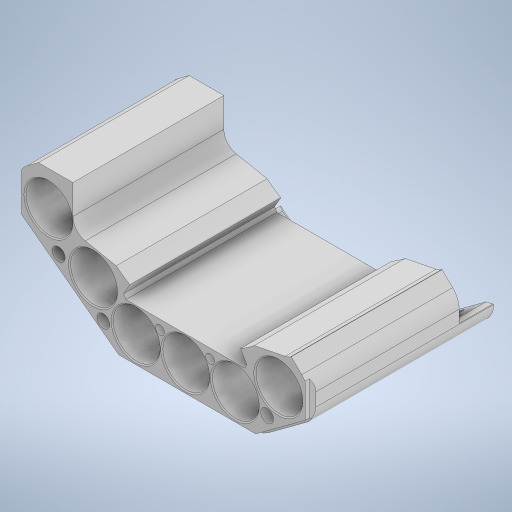
# Autodesk Inventor part: battery_mnt_right
Saved by Autodesk Inventor 2023.4 (Build 274418000, 418)
## iProperties
Created: 2024-01-27
Part Number: battery_mnt_right
Material: Generic
Document SubType Name: Modeling
Designer: aaron
Density: 1 g/cm^3
Appearance: Default
Author: aaron
Autodesk Inventor part; units mm, degrees
ref_plane "YZ Plane" through (0, 0, 0) normal (1, 0, 0) x (0, 1, 0)
ref_plane "XZ Plane" through (0, 0, 0) normal (0, 1, 0) x (-1, 0, 0)
ref_plane "XY Plane" through (0, 0, 0) normal (0, 0, 1) x (1, 0, 0)
sketch "Sketch1" plane through (0, 0, 0) normal (0, 0, 1) x (1, 0, 0)
  line L0 (28.444864, -49.267949) -> (27.444864, -51)
  line L1 (28.444864, -49.267949) -> (25.5, -44.167296)
  arc A0 (25.5, -44.167296) -> (38.751507, -33.156006) centre (0, 0) ccw
  arc A1 (38.751507, -33.156006) -> (51.999677, -30) centre (44.999677, -30) ccw
  line L2 (51.999677, 30) -> (51.999677, -30)
  arc A2 (51.999677, 30) -> (38.751507, 33.156006) centre (44.999677, 30) ccw
  arc A3 (38.751507, 33.156006) -> (25.5, 44.167296) centre (0, 0) ccw
  line L3 (25.5, 44.167296) -> (28.444864, 49.267949)
  line L4 (27.444864, 51) -> (28.444864, 49.267949)
  line L5 (27.444864, 51) -> (-27.444864, 51)
  line L6 (-28.444864, 49.267949) -> (-27.444864, 51)
  line L7 (-28.444864, 49.267949) -> (-25.5, 44.167296)
  arc A4 (-25.5, 44.167296) -> (-38.751507, 33.156006) centre (0, 0) ccw
  arc A5 (-38.751507, 33.156006) -> (-51.999677, 30) centre (-44.999677, 30) ccw
  line L8 (-51.999677, 30) -> (-51.999677, -30)
  arc A6 (-51.999677, -30) -> (-38.751507, -33.156006) centre (-44.999677, -30) ccw
  arc A7 (-38.751507, -33.156006) -> (-25.5, -44.167296) centre (0, 0) ccw
  line L9 (-25.5, -44.167296) -> (-28.444864, -49.267949)
  line L10 (-27.444864, -51) -> (-28.444864, -49.267949)
  line L11 (-27.444864, -51) -> (27.444864, -51)
  circle A8 centre (0, 0) radius 48
  circle A9 centre (44.999677, -30) radius 2.875
  circle A10 centre (44.999677, 30) radius 2.875
  circle A11 centre (-44.999677, 30) radius 2.875
  circle A12 centre (-44.999677, -30) radius 2.875
  line L12 (-43.944685, -76.472384) -> (38.141017, -76.472384)
  circle A13 centre (43.188005, -51) radius 10.85
  circle A14 centre (23, -63) radius 10.85
  circle A15 centre (0, -63) radius 10.85
  circle A16 centre (-23, -63) radius 10.85
  circle A17 centre (-63.495945, -32.562911) radius 10.85
  circle A18 centre (-42.787465, -50.133975) radius 10.85
  line L13 (-51.999677, -16.395024) -> (-68.142845, -16.395024)
  line L14 (57.082969, -58.824434) -> (57.082969, -43.439377)
  line L15 (57.082969, -43.439377) -> (49.113739, -35.663435)
  line L16 (-77.442937, -41.876031) -> (-31.413941, -76.472384)
  line L17 (57.082969, -58.824434) -> (33.195718, -76.472384)
  line L18 (-77.442937, -41.876031) -> (-77.442937, -23.26595)
  line L19 (-77.442937, -23.26595) -> (-68.142845, -16.395024)
  line L20 (-47.70661, -36.599635) -> (-27.043212, -40.695389)
  line L21 (0, 0) -> (0, -13.401061)
  line L22 (47.70661, -36.599635) -> (27.043212, -40.695389)
  point P0 (-43.377516, -36.809449)
  point P1 (43.377516, -36.809449)
  point P2 (-31.997646, -39.713356)
  point P3 (-46.360689, -36.866414)
  point P4 (46.360689, -36.866414)
  point P5 (31.997646, -39.713356)
  dimension "d2" = 21.7
  dimension "d3" = 21.7
  dimension "d4" = 21.7
  dimension "d5" = 21.7
  dimension "d6" = 21.7
  dimension "d7" = 21.7
  dimension "d12" = 96
  dimension "d13" = 54.88973
  dimension "d14" = 54.88973
  dimension "d15" = 60
  dimension "d16" = 60
  dimension "d17" = 7
  dimension "d18" = 7
  dimension "d19" = 51
  dimension "d20" = 51
  dimension "d21" = 12
  dimension "d22" = 12
  dimension "d23" = 12
  dimension "d24" = 23
  dimension "d25" = 0
  dimension "d26" = 23
  dimension "d28" = 102
  dimension "d29" = 51
  constraints: 46 end point, 19 centre point, 19 point on circle, 3 point on line, 2 symmetric about line, 2 vertical, 1 horizontal, 1 perpendicular, 1 tangent
  measures "d2" diameter of A13
  measures "d3" diameter of A14
  measures "d4" diameter of A15
  measures "d5" diameter of A16
  measures "d6" diameter of A17
  measures "d7" diameter of A18
  measures "d12" diameter of A8
  measures "d13" distance of L11.start L0.end
  measures "d14" distance of L5.start L6.end
  measures "d15" distance of L8.start L8.end
  measures "d16" distance of L2.start L2.end
  measures "d17" radius of A1
  measures "d18" radius of A6
  measures "d19" radius of A7
  measures "d20" radius of A0
  measures "d21" distance from line of A15.centre L11
  measures "d22" distance from line of L11 A14.centre
  measures "d23" distance from line of L11 A16.centre
  measures "d24" distance of A16.centre A15.centre
  measures "d25" horizontal distance of point (0, 0) A15.centre
  measures "d26" distance of A15.centre A14.centre
  measures "d28" distance between parallel lines of L5 L11
  measures "d29" distance from line of point (0, 0) L11
extrude "Extrusion1" add sketch "Sketch1" along normal blind 70 contours L1 A0 L22 A1 L15 L14 L17 L12 L16 L18 L19 L13 L8 A6 L20 A7 L9 L10 L11 L0
thicken "Thicken1" operation cut thickness 0.1 both sides no extend neighbours no toward (-1, 0, 0) faces at (-51.999677, -25.465008, 23.333333) (-51.022382, -33.567495, 46.666667) (-31.310695, -40.257178, 46.666667) (-27.463242, -47.567731, 23.333333) (-27.778197, -50.42265, 23.333333) (9.148288, -51, 23.333333) (28.11153, -49.845299, 23.333333) (26.481621, -45.867513, 23.333333) (31.310695, -40.257178, 23.333333) (48.836892, -35.854552, 23.333333) (-36.785327, -38.764375, 46.666667) (41.573008, -37.815395, 23.333333)
sketch "Sketch2" plane through (0, 0, 0) normal (0, 0, -1) x (-1, 0, 0)
  line L0 (-49.172511, -35.744341) -> (-49.113739, -35.663435)
  line L1 (-57.082969, -43.439377) -> (-49.113739, -35.663435)
  line L2 (-57.082969, -58.824434) -> (-57.082969, -43.439377)
  line L3 (-33.195718, -76.472384) -> (-57.082969, -58.824434)
  line L4 (31.413941, -76.472384) -> (-33.195718, -76.472384)
  line L5 (77.442937, -41.876031) -> (31.413941, -76.472384)
  line L6 (77.442937, -23.26595) -> (77.442937, -41.876031)
  line L7 (68.142845, -16.395024) -> (77.442937, -23.26595)
  line L8 (52.099677, -16.395024) -> (68.142845, -16.395024)
  line L9 (52.099677, -16.395024) -> (52.099677, -30)
  arc A0 (46.380132, -36.964506) -> (52.099677, -30) centre (44.999677, -30) ccw
  line L10 (46.380132, -36.964506) -> (32.041213, -39.806666)
  arc A1 (25.636554, -44.203813) -> (32.041213, -39.806666) centre (0, 0) ccw
  line L11 (25.636554, -44.203813) -> (28.560334, -49.267949)
  line L12 (28.560334, -49.267949) -> (27.502599, -51.1)
  line L13 (27.502599, -51.1) -> (-27.502599, -51.1)
  line L14 (-27.502599, -51.1) -> (-28.560334, -49.267949)
  line L15 (-28.560334, -49.267949) -> (-25.636554, -44.203813)
  arc A2 (-32.041213, -39.806666) -> (-25.636554, -44.203813) centre (0, 0) ccw
  line L16 (-32.041213, -39.806666) -> (-46.380132, -36.964506)
  arc A3 (-49.172511, -35.744341) -> (-46.380132, -36.964506) centre (-44.999677, -30) ccw
  circle A4 centre (0, -63) radius 10.85
  circle A5 centre (42.787465, -50.133975) radius 10.85
  circle A6 centre (63.495945, -32.562911) radius 10.85
  circle A7 centre (23, -63) radius 10.85
  circle A8 centre (-23, -63) radius 10.85
  circle A9 centre (-43.188005, -51) radius 10.85
  line L17 (-63.021311, -52.572205) -> (-32.701715, -74.972384)
  line L18 (-32.701715, -74.972384) -> (30.913077, -74.972384)
  line L19 (30.913077, -74.972384) -> (84.461316, -34.724411)
  line L20 (-33.195718, -76.472384) -> (-57.082969, -58.824434)
  line L21 (-55.582969, -67.648409) -> (-55.582969, -26.578043)
  line L22 (75.942937, -58.824434) -> (75.942937, -10.568938)
  point P0 (77.442937, -39.999571)
  point P1 (-57.082969, -56.959464)
  point P2 (75.942937, -22.157747)
  point P3 (75.942937, -41.127002)
  point P4 (-55.582969, -58.067667)
  point P5 (-55.582969, -41.975759)
  dimension "d30" = 1.5
  dimension "d32" = 1.5
  dimension "d33" = 1.5
  dimension "d50" = 1.5
  dimension "d51" = 1.5
  constraints: 10 end point, 2 vertical, 1 horizontal, 1 parallel
  measures "d30" distance between parallel lines of L4 L18
  measures "d32" distance between parallel lines of L3 L17
  measures "d33" distance between parallel lines of L5 L19
  measures "d50" distance between parallel lines of L6 L22
  measures "d51" distance between parallel lines of L2 L21
extrude "Extrusion2" cut sketch "Sketch2" against normal blind 2 contours L21 L17 L2 L1 | L21 L3 L2 L17 | L17 L18 L19 L22 L5 L4 L3 L21 | L22 L7 L6 L19 | L19 L6 L5 L22
sketch "Sketch3" plane through (0, 0, 0) normal (0, 0, -1) x (-1, 0, 0)
  circle A0 centre (38, -64.972384) radius 2.95
  circle A1 centre (-38, -64.972384) radius 2.95
  circle A2 centre (0, -63) radius 10.85
  line L0 (31.413941, -76.472384) -> (-33.195718, -76.472384)
  circle A3 centre (58.715512, -48.446115) radius 2.95
  line L1 (77.442937, -41.876031) -> (31.413941, -76.472384)
  point P0 (0, 0)
  dimension "d36" = 5.9
  dimension "d37" = 5.9
  dimension "d38" = 38
  dimension "d39" = 38
  dimension "d40" = 11.5
  dimension "d41" = 11.5
  dimension "d44" = 5.9
  dimension "d45" = 26.5
  dimension "d46" = 6
  constraints: 3 centre point
  measures "d36" diameter of A1
  measures "d37" diameter of A0
  measures "d38" horizontal distance of A1.centre A2.centre
  measures "d39" horizontal distance of A0.centre A2.centre
  measures "d40" distance from line of L0 A0.centre
  measures "d41" distance from line of L0 A1.centre
  measures "d44" diameter of A3
  measures "d45" distance of A0.centre A3.centre
  measures "d46" distance from line of L1 A3.centre
extrude "Extrusion3" cut sketch "Sketch3" against normal blind 15 contours A0 | A1 | A3
chamfer "Chamfer1" distance 1.5 angle 45 5 edges at (45.1393, -67.6484, 2) (0.8909, -76.4724, 2) (-54.4284, -59.1742, 2) (-77.4429, -32.571, 2) (57.083, -51.1319, 2)
sketch "Sketch4" plane through (0, 0, 70) normal (0, 0, 1) x (1, 0, 0)
  circle A0 centre (43.188005, -51) radius 10.85
  circle A1 centre (23, -63) radius 10.85
  circle A2 centre (-23, -63) radius 10.85
  circle A3 centre (-63.495945, -32.562911) radius 10.85
  circle A4 centre (-42.787465, -50.133975) radius 10.85
  circle A5 centre (0, -63) radius 10.85
  line L0 (49.113739, -35.663435) -> (49.172511, -35.744341)
  arc A6 (46.380132, -36.964506) -> (49.172511, -35.744341) centre (44.999677, -30) ccw
  line L1 (46.380132, -36.964506) -> (32.041213, -39.806666)
  arc A7 (25.636554, -44.203813) -> (32.041213, -39.806666) centre (0, 0) ccw
  line L2 (25.636554, -44.203813) -> (28.560334, -49.267949)
  line L3 (28.560334, -49.267949) -> (27.502599, -51.1)
  line L4 (27.502599, -51.1) -> (-27.502599, -51.1)
  line L5 (-27.502599, -51.1) -> (-28.560334, -49.267949)
  line L6 (-28.560334, -49.267949) -> (-25.636554, -44.203813)
  arc A8 (-32.041213, -39.806666) -> (-25.636554, -44.203813) centre (0, 0) ccw
  line L7 (-32.041213, -39.806666) -> (-46.380132, -36.964506)
  arc A9 (-52.099677, -30) -> (-46.380132, -36.964506) centre (-44.999677, -30) ccw
  line L8 (-52.099677, -30) -> (-52.099677, -16.395024)
  line L9 (-52.099677, -16.395024) -> (-68.142845, -16.395024)
  line L10 (-68.142845, -16.395024) -> (-77.442937, -23.26595)
  line L11 (-77.442937, -23.26595) -> (-77.442937, -41.876031)
  line L12 (-77.442937, -41.876031) -> (-31.413941, -76.472384)
  line L13 (-31.413941, -76.472384) -> (33.195718, -76.472384)
  line L14 (33.195718, -76.472384) -> (57.082969, -58.824434)
  line L15 (57.082969, -58.824434) -> (57.082969, -43.439377)
  line L16 (57.082969, -43.439377) -> (49.113739, -35.663435)
  line L17 (-77.442937, -23.26595) -> (-77.442937, -41.876031)
  line L18 (-77.442937, -34.370192) -> (-29.410485, -70.472384)
  line L19 (-29.410485, -70.472384) -> (31.219707, -70.472384)
  line L20 (31.219707, -70.472384) -> (83.321801, -31.979251)
  line L21 (-40.549713, -62.099908) -> (-46.975634, -69.813396)
  point P0 (57.082969, -51.364553)
  point P1 (-65.717928, -43.182953)
  point P2 (-73.079596, -37.64977)
  point P3 (-42.066335, -60.959984)
  point P4 (-53.387176, -52.451003)
  point P5 (-44.394934, -66.715599)
  dimension "d65" = 6
  dimension "d66" = 6
  dimension "d67" = 6
  constraints: 8 end point, 3 parallel, 2 point on line, 1 horizontal
  measures "d65" distance between parallel lines of L13 L19
  measures "d66" distance between parallel lines of L14 L20
  measures "d67" distance between parallel lines of L12 L18
extrude "Extrusion4" add sketch "Sketch4" along normal blind 16 contours L20 A0 | A0 L20 L15 L14 L13 L12 L21 L18 A2 L19 A5 A1 | A1 L19 | A5 L19 | A2 L18 L19 picked at (49.762113, -57.29404) picked at (21.019918, -71.008065) picked at (1.980082, -71.008065) picked at (-20.549607, -71.0179)
chamfer "Chamfer2" distance 0.5 angle 45 6 edges at (32.338, -51, 0) (12.15, -63, 0) (-10.85, -63, 0) (-33.85, -63, 0) (-53.6375, -50.134, 0) (-74.3459, -32.5629, 0)
sketch "Sketch6" plane through (-40.549713, -62.099908, 86) normal (0.6008289, 0.7993777, 0) x (0.7993777, -0.6008289, 0)
  circle A0 centre (7.934875, 6) radius 1.65
  line L0 (13.934875, 0) -> (0, 0)
  line L1 (13.934875, 16) -> (13.934875, 0)
  point P0 (-4.896886, 86)
  dimension "d68" = 3.3
  dimension "d69" = 6
  dimension "d70" = 6
  constraints: 1 centre point
  measures "d68" diameter of A0
  measures "d69" distance from line of L0 A0.centre
  measures "d70" distance from line of L1 A0.centre
extrude "Extrusion6" cut sketch "Sketch6" against normal through all
sketch "Sketch7" plane through (15.133236, -70.472384, 70) normal (0, 1, 0) x (1, 0, 0)
  circle A0 centre (-32.543721, -10) radius 1.65
  circle A1 centre (4.086471, -10) radius 1.65
  line L0 (16.086471, -16) -> (-44.543721, -16)
  line L1 (-44.543721, 0) -> (-44.543721, -16)
  line L2 (16.086471, 0) -> (16.086471, -16)
  point P0 (-15.133236, 70)
  dimension "d73" = 6
  dimension "d74" = 3.3
  dimension "d75" = 3.3
  dimension "d76" = 6
  dimension "d77" = 12
  dimension "d78" = 12
  constraints: 2 centre point
  measures "d73" distance from line of L0 A0.centre
  measures "d74" diameter of A0
  measures "d75" diameter of A1
  measures "d76" distance from line of L0 A1.centre
  measures "d77" distance from line of L1 A0.centre
  measures "d78" distance from line of L2 A1.centre
extrude "Extrusion7" cut sketch "Sketch7" against normal through all
sketch "Sketch8" plane through (31.219707, -70.472384, 86) normal (-0.5942202, 0.8043024, 0) x (0.8043024, 0.5942202, 0)
  circle A0 centre (20.156143, 6) radius 1.65
  line L0 (32.156143, 16) -> (32.156143, 0)
  line L1 (32.156143, 0) -> (0, 0)
  point P0 (16.766032, 86)
  dimension "d81" = 3.3
  dimension "d82" = 12
  dimension "d83" = 6
  constraints: 1 centre point
  measures "d81" diameter of A0
  measures "d82" distance from line of L0 A0.centre
  measures "d83" distance from line of L1 A0.centre
extrude "Extrusion8" cut sketch "Sketch8" against normal through all
sketch "Sketch9" plane through (-31.413941, -76.472384, 3.5) normal (-0.6008289, -0.7993777, 0) x (0.7993777, -0.6008289, 0)
  circle A0 centre (-8.003456, 76.5) radius 1.65
  circle A1 centre (-8.003456, 76.5) radius 1.65
  circle A2 centre (-8.003456, 76.5) radius 2.65
  point P0 (-20.835216, -3.5)
  dimension "d86" = 5.3
  constraints: 1 centre point, 1 coincident
  measures "d86" diameter of A2
extrude "Extrusion9" cut sketch "Sketch9" against normal blind 3 contours A0 | A2
sketch "Sketch10" plane through (-31.413941, -76.472384, 3.5) normal (0, -1, 0) x (1, 0, 0)
  circle A0 centre (14.003456, 76.5) radius 1.65
  circle A1 centre (14.003456, 76.5) radius 2.65
  circle A2 centre (50.633647, 76.5) radius 1.65
  circle A3 centre (50.633647, 76.5) radius 2.65
  point P0 (31.413941, -3.5)
  dimension "d89" = 5.3
  dimension "d90" = 5.3
  constraints: 2 centre point, 2 coincident
  measures "d89" diameter of A1
  measures "d90" diameter of A3
extrude "Extrusion10" cut sketch "Sketch10" against normal blind 3 contours A0 | A1 | A2 | A3
sketch "Sketch11" plane through (57.082969, -58.824434, 3.5) normal (0.5942202, -0.8043024, 0) x (0.8043024, 0.5942202, 0)
  circle A0 centre (-7.567188, 76.5) radius 1.65
  circle A1 centre (-7.567188, 76.5) radius 2.65
  point P0 (-10.957298, -3.5)
  dimension "d93" = 5.3
  constraints: 1 centre point, 1 coincident
  measures "d93" diameter of A1
extrude "Extrusion11" cut sketch "Sketch11" against normal blind 3
fillet "Fillet1" radius 10 6 edges at (-31.4139, -76.4724, 44.7499) (33.1957, -76.4724, 44.7499) (57.083, -58.8244, 44.7499) (57.083, -43.4394, 36.7499) (-77.4429, -41.876, 36.7499) (-77.4429, -23.266, 36.7499)
chamfer "Chamfer5" distance 2 angle 45 6 edges at (0.9046, -70.4724, 86) (44.1513, -60.9185, 86) (-34.9801, -66.2861, 86) (-40.5497, -62.0999, 78) (-44.3949, -66.7156, 78) (57.083, -51.3646, 78)
mirror "Mirror1" about plane through (-10.179984, -46.433704, 0) normal (0, 0, -1) remove original yes
sketch "Sketch16" plane through (-68.142845, -16.395024, 0) normal (0, 0, 1) x (1, 0, 0)
  circle A0 centre (56.431219, -38.970604) radius 2
  circle A1 centre (79.685977, -38.970604) radius 2
  point P0 (68.142845, 16.395024)
  dimension "d105" = 4
  dimension "d106" = 4
  constraints: 2 centre point
  measures "d105" diameter of A0
  measures "d106" diameter of A1
extrude "Extrusion13" cut sketch "Sketch16" against normal through all
equation "\"d2\" = d6"
equation "\"d3\" = d6"
equation "\"d4\" = d6"
equation "\"d5\" = d6"
equation "\"d7\" = d6"
equation "\"d22\" = d21"
equation "\"d23\" = d21"
equation "\"d26\" = d24"
body "Solid1"
